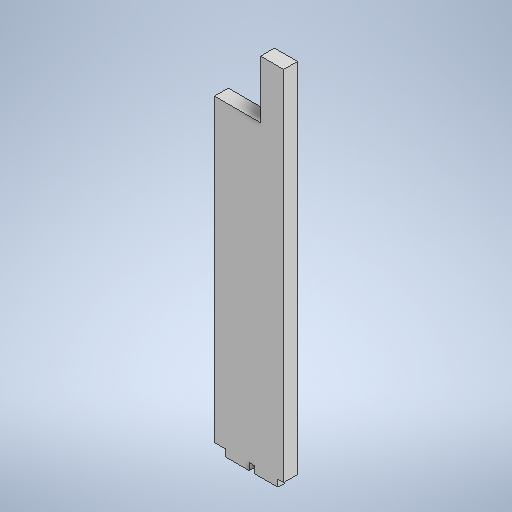
# Autodesk Inventor part: Archimedes Screw Border3
Saved by Autodesk Inventor 2025.3 (Build 293356000, 356)
## iProperties
Created: 2026-04-08
Part Number: Archimedes Screw Border3
Material: Generic
Document SubType Name: Modeling
Designer: ziada
Density: 1 g/cm^3
Appearance: Default
Author: ziada
Autodesk Inventor part; units mm, degrees
ref_plane "YZ Plane" through (0, 0, 0) normal (1, 0, 0) x (0, 1, 0)
ref_plane "XZ Plane" through (0, 0, 0) normal (0, 1, 0) x (-1, 0, 0)
ref_plane "XY Plane" through (0, 0, 0) normal (0, 0, 1) x (1, 0, 0)
sketch "Sketch1" plane through (0, 0, 0) normal (0, 0, 1) x (1, 0, 0)
  line L0 (0, 266) -> (0, 6)
  line L1 (60, 6) -> (60, 316)
  line L2 (0, 6) -> (10, 6)
  line L3 (10, 6) -> (10, 0)
  line L4 (10, 0) -> (30, 0)
  line L5 (30, 0) -> (30, 6)
  line L6 (30, 6) -> (35, 6)
  line L7 (35, 6) -> (35, 0)
  line L8 (35, 0) -> (55, 0)
  line L9 (55, 0) -> (55, 6)
  line L10 (55, 6) -> (60, 6)
  line L11 (60, 316) -> (40, 316)
  line L12 (40, 316) -> (40, 266)
  line L13 (40, 266) -> (0, 266)
  point P0 (0, 0)
  dimension "d25" = 10
  dimension "d26" = 20
  dimension "d27" = 5
  dimension "d29" = 20
  dimension "d31" = 310
  dimension "d32" = 20
  dimension "d33" = 50
  dimension "d34" = 6
  constraints: 28 end point, 7 perpendicular, 3 horizontal, 3 point on line, 2 parallel, 1 vertical
  measures "d25" distance of L0.end L2.end
  measures "d26" distance of L3.end L4.end
  measures "d27" distance of L5.end L6.end
  measures "d29" distance of L7.end L8.end
  measures "d31" distance of L1.start L1.end
  measures "d32" distance of L1.end L11.end
  measures "d33" distance of L11.end L12.end
  measures "d34" distance of L2.end L3.end
extrude "Extrusion1" add sketch "Sketch1" against normal blind 6
sketch "Sketch3" plane through (0, 0, -6) normal (0, 0, -1) x (-1, 0, 0)
  line L0 (-60, 316) -> (-60, 6) projected
  line L1 (-60, 316) -> (-60, 6)
  line L2 (-60, 6) -> (0, 6)
  line L3 (-40, 316) -> (-60, 316)
  line L4 (0, 6) -> (0, 266) projected
  line L5 (0, 6) -> (0, 266)
  line L6 (0, 266) -> (-40, 266)
  line L7 (-40, 266) -> (-40, 316) projected
  line L8 (-40, 266) -> (-40, 316)
  point P0 (0, 0)
  constraints: 12 end point, 2 collinear, 2 perpendicular, 1 vertical
extrude "Extrusion3" add sketch "Sketch3" along normal blind 6
body "Solid1"
